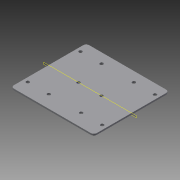
# Autodesk Inventor part: piastra_manicotti
Saved by Autodesk Inventor 2014 SP1 (Build 180222100, 222)
## iProperties
Created: 2015-04-08
Part Number: piastra_manicotti
Material: Generic
Document SubType Name: Modeling
Designer: Giorgio Nuzzo
Density: 1 g/cm^3
Appearance: Default
d2: 4,000 mm
d3: 2,000 mm
d4: 0,00 deg
d5: 4,200 mm
d6: 15,000 mm
d7: 4,200 mm
d8: 5,500 mm
d9: 12,900 mm
d10: 4,200 mm
d11: 27,400 mm
d12: 12,900 mm
d13: 2,000 mm
d14: 0,00 deg
Author: Giorgio Nuzzo
Autodesk Inventor part; units mm, degrees
ref_plane "YZ Plane" through (0, 0, 0) normal (1, 0, 0) x (0, 1, 0)
ref_plane "XZ Plane" through (0, 0, 0) normal (0, 1, 0) x (-1, 0, 0)
ref_plane "XY Plane" through (0, 0, 0) normal (0, 0, 1) x (1, 0, 0)
sketch "Sketch1" plane through (0, 0, 0) normal (0, 0, 1) x (1, 0, 0)
  line L0 (0, 69.8302) -> (0, -69.8234) construction
  line L1 (-76.7674, 0) -> (76.7472, 0) construction
  line L2 (-17.1109, 0.0005) -> (-17.1001, 0.2151)
  line L3 (-17.1001, 0.2151) -> (-17.0684, 0.4237)
  line L4 (-17.0684, 0.4237) -> (-17.0166, 0.6249)
  line L5 (-17.0166, 0.6249) -> (-16.9459, 0.8178)
  line L6 (-16.9459, 0.8178) -> (-16.8576, 1.0014)
  line L7 (-16.8576, 1.0014) -> (-16.7523, 1.1745)
  line L8 (-16.7523, 1.1745) -> (-16.6314, 1.3361)
  line L9 (-16.6314, 1.3361) -> (-16.496, 1.4853)
  line L10 (-16.496, 1.4853) -> (-16.3468, 1.6209)
  line L11 (-16.3468, 1.6209) -> (-16.1851, 1.7418)
  line L12 (-16.1851, 1.7418) -> (-16.012, 1.8469)
  line L13 (-16.012, 1.8469) -> (-15.8285, 1.9354)
  line L14 (-15.8285, 1.9354) -> (-15.6354, 2.006)
  line L15 (-15.6354, 2.006) -> (-15.4342, 2.0577)
  line L16 (-15.4342, 2.0577) -> (-15.2258, 2.0896)
  line L17 (-15.2258, 2.0896) -> (-15.011, 2.1004)
  line L18 (-15.011, 2.1004) -> (-14.7964, 2.0896)
  line L19 (-14.7964, 2.0896) -> (-14.5878, 2.0577)
  line L20 (-14.5878, 2.0577) -> (-14.3866, 2.006)
  line L21 (-14.3866, 2.006) -> (-14.1936, 1.9354)
  line L22 (-14.1936, 1.9354) -> (-14.01, 1.8469)
  line L23 (-14.01, 1.8469) -> (-13.8369, 1.7418)
  line L24 (-13.8369, 1.7418) -> (-13.6752, 1.6209)
  line L25 (-13.6752, 1.6209) -> (-13.5262, 1.4853)
  line L26 (-13.5262, 1.4853) -> (-13.3906, 1.3361)
  line L27 (-13.3906, 1.3361) -> (-13.2697, 1.1745)
  line L28 (-13.2697, 1.1745) -> (-13.1644, 1.0014)
  line L29 (-13.1644, 1.0014) -> (-13.0761, 0.8178)
  line L30 (-13.0761, 0.8178) -> (-13.0054, 0.6249)
  line L31 (-13.0054, 0.6249) -> (-12.9537, 0.4237)
  line L32 (-12.9537, 0.4237) -> (-12.9219, 0.2151)
  line L33 (-12.9219, 0.2151) -> (-12.911, 0.0005)
  line L34 (-12.911, 0.0005) -> (-12.9219, -0.2143)
  line L35 (-12.9219, -0.2143) -> (-12.9537, -0.4228)
  line L36 (-12.9537, -0.4228) -> (-13.0054, -0.624)
  line L37 (-13.0054, -0.624) -> (-13.0761, -0.8169)
  line L38 (-13.0761, -0.8169) -> (-13.1644, -1.0005)
  line L39 (-13.1644, -1.0005) -> (-13.2697, -1.1738)
  line L40 (-13.2697, -1.1738) -> (-13.3906, -1.3354)
  line L41 (-13.3906, -1.3354) -> (-13.5262, -1.4846)
  line L42 (-13.5262, -1.4846) -> (-13.6752, -1.6199)
  line L43 (-13.6752, -1.6199) -> (-13.8369, -1.7409)
  line L44 (-13.8369, -1.7409) -> (-14.01, -1.8463)
  line L45 (-14.01, -1.8463) -> (-14.1936, -1.9345)
  line L46 (-14.1936, -1.9345) -> (-14.3866, -2.0051)
  line L47 (-14.3866, -2.0051) -> (-14.5878, -2.0568)
  line L48 (-14.5878, -2.0568) -> (-14.7964, -2.0888)
  line L49 (-14.7964, -2.0888) -> (-15.011, -2.0995)
  line L50 (-15.011, -2.0995) -> (-15.2258, -2.0888)
  line L51 (-15.2258, -2.0888) -> (-15.4342, -2.0568)
  line L52 (-15.4342, -2.0568) -> (-15.6354, -2.0051)
  line L53 (-15.6354, -2.0051) -> (-15.8285, -1.9345)
  line L54 (-15.8285, -1.9345) -> (-16.012, -1.8463)
  line L55 (-16.012, -1.8463) -> (-16.1851, -1.7409)
  line L56 (-16.1851, -1.7409) -> (-16.3468, -1.6199)
  line L57 (-16.3468, -1.6199) -> (-16.496, -1.4846)
  line L58 (-16.496, -1.4846) -> (-16.6314, -1.3354)
  line L59 (-16.6314, -1.3354) -> (-16.7523, -1.1738)
  line L60 (-16.7523, -1.1738) -> (-16.8576, -1.0005)
  line L61 (-16.8576, -1.0005) -> (-16.9459, -0.8169)
  line L62 (-16.9459, -0.8169) -> (-17.0166, -0.624)
  line L63 (-17.0166, -0.624) -> (-17.0684, -0.4228)
  line L64 (-17.0684, -0.4228) -> (-17.1001, -0.2143)
  line L65 (-17.1001, -0.2143) -> (-17.1109, 0.0005)
  spline S0 degree 3 poles (-53.96, -44.9961) (-53.96, -47.2051) (-52.1691, -48.9962) (-49.9599, -48.9962) knots 0 0 0 0 1 1 1 1
  line L66 (-53.96, -44.9961) -> (-53.96, -47.2051) construction
  line L67 (-53.96, -47.2051) -> (-52.1691, -48.9962) construction
  line L68 (-52.1691, -48.9962) -> (-49.9599, -48.9962) construction
  line L69 (-49.9599, -48.9962) -> (49.9401, -48.9962)
  spline S1 degree 3 poles (49.9401, -48.9962) (52.1491, -48.9962) (53.9398, -47.2051) (53.9398, -44.9961) knots 2 2 2 2 3 3 3 3
  line L70 (49.9401, -48.9962) -> (52.1491, -48.9962) construction
  line L71 (52.1491, -48.9962) -> (53.9398, -47.2051) construction
  line L72 (53.9398, -47.2051) -> (53.9398, -44.9961) construction
  line L73 (53.9398, -44.9961) -> (53.9398, 45.0029)
  spline S2 degree 3 poles (53.9398, 45.0029) (53.9398, 47.212) (52.1491, 49.003) (49.9401, 49.003) knots 4 4 4 4 5 5 5 5
  line L74 (53.9398, 45.0029) -> (53.9398, 47.212) construction
  line L75 (53.9398, 47.212) -> (52.1491, 49.003) construction
  line L76 (52.1491, 49.003) -> (49.9401, 49.003) construction
  line L77 (49.9401, 49.003) -> (-49.9599, 49.003)
  spline S3 degree 3 poles (-49.9599, 49.003) (-52.1691, 49.003) (-53.96, 47.212) (-53.96, 45.0029) knots 6 6 6 6 7 7 7 7
  line L78 (-49.9599, 49.003) -> (-52.1691, 49.003) construction
  line L79 (-52.1691, 49.003) -> (-53.96, 47.212) construction
  line L80 (-53.96, 47.212) -> (-53.96, 45.0029) construction
  line L81 (-53.96, 45.0029) -> (-53.96, -44.9961)
  line L82 (39.7398, -16.7966) -> (39.7516, -16.5665)
  line L83 (39.7516, -16.5665) -> (39.7857, -16.3432)
  line L84 (39.7857, -16.3432) -> (39.8411, -16.1276)
  line L85 (39.8411, -16.1276) -> (39.9169, -15.9209)
  line L86 (39.9169, -15.9209) -> (40.0117, -15.7242)
  line L87 (40.0117, -15.7242) -> (40.1243, -15.5385)
  line L88 (40.1243, -15.5385) -> (40.2539, -15.3655)
  line L89 (40.2539, -15.3655) -> (40.3989, -15.2057)
  line L90 (40.3989, -15.2057) -> (40.5587, -15.0603)
  line L91 (40.5587, -15.0603) -> (40.732, -14.9308)
  line L92 (40.732, -14.9308) -> (40.9174, -14.8181)
  line L93 (40.9174, -14.8181) -> (41.1141, -14.7234)
  line L94 (41.1141, -14.7234) -> (41.3208, -14.6479)
  line L95 (41.3208, -14.6479) -> (41.5365, -14.5925)
  line L96 (41.5365, -14.5925) -> (41.7601, -14.5583)
  line L97 (41.7601, -14.5583) -> (41.9898, -14.5466)
  line L98 (41.9898, -14.5466) -> (42.22, -14.5583)
  line L99 (42.22, -14.5583) -> (42.4436, -14.5925)
  line L100 (42.4436, -14.5925) -> (42.6592, -14.6479)
  line L101 (42.6592, -14.6479) -> (42.8659, -14.7234)
  line L102 (42.8659, -14.7234) -> (43.0626, -14.8181)
  line L103 (43.0626, -14.8181) -> (43.248, -14.9308)
  line L104 (43.248, -14.9308) -> (43.4213, -15.0603)
  line L105 (43.4213, -15.0603) -> (43.5811, -15.2057)
  line L106 (43.5811, -15.2057) -> (43.7262, -15.3655)
  line L107 (43.7262, -15.3655) -> (43.8557, -15.5385)
  line L108 (43.8557, -15.5385) -> (43.9684, -15.7242)
  line L109 (43.9684, -15.7242) -> (44.0631, -15.9209)
  line L110 (44.0631, -15.9209) -> (44.1389, -16.1276)
  line L111 (44.1389, -16.1276) -> (44.1944, -16.3432)
  line L112 (44.1944, -16.3432) -> (44.2285, -16.5665)
  line L113 (44.2285, -16.5665) -> (44.2398, -16.7966)
  line L114 (44.2398, -16.7966) -> (44.2285, -17.0268)
  line L115 (44.2285, -17.0268) -> (44.1944, -17.25)
  line L116 (44.1944, -17.25) -> (44.1389, -17.4657)
  line L117 (44.1389, -17.4657) -> (44.0631, -17.6724)
  line L118 (44.0631, -17.6724) -> (43.9684, -17.8691)
  line L119 (43.9684, -17.8691) -> (43.8557, -18.0548)
  line L120 (43.8557, -18.0548) -> (43.7262, -18.2277)
  line L121 (43.7262, -18.2277) -> (43.5811, -18.3876)
  line L122 (43.5811, -18.3876) -> (43.4213, -18.533)
  line L123 (43.4213, -18.533) -> (43.248, -18.6625)
  line L124 (43.248, -18.6625) -> (43.0626, -18.7751)
  line L125 (43.0626, -18.7751) -> (42.8659, -18.8699)
  line L126 (42.8659, -18.8699) -> (42.6592, -18.9453)
  line L127 (42.6592, -18.9453) -> (42.4436, -19.0008)
  line L128 (42.4436, -19.0008) -> (42.22, -19.0349)
  line L129 (42.22, -19.0349) -> (41.9898, -19.0466)
  line L130 (41.9898, -19.0466) -> (41.7601, -19.0349)
  line L131 (41.7601, -19.0349) -> (41.5365, -19.0008)
  line L132 (41.5365, -19.0008) -> (41.3208, -18.9453)
  line L133 (41.3208, -18.9453) -> (41.1141, -18.8699)
  line L134 (41.1141, -18.8699) -> (40.9174, -18.7751)
  line L135 (40.9174, -18.7751) -> (40.732, -18.6625)
  line L136 (40.732, -18.6625) -> (40.5587, -18.533)
  line L137 (40.5587, -18.533) -> (40.3989, -18.3876)
  line L138 (40.3989, -18.3876) -> (40.2539, -18.2277)
  line L139 (40.2539, -18.2277) -> (40.1243, -18.0548)
  line L140 (40.1243, -18.0548) -> (40.0117, -17.8691)
  line L141 (40.0117, -17.8691) -> (39.9169, -17.6724)
  line L142 (39.9169, -17.6724) -> (39.8411, -17.4657)
  line L143 (39.8411, -17.4657) -> (39.7857, -17.25)
  line L144 (39.7857, -17.25) -> (39.7516, -17.0268)
  line L145 (39.7516, -17.0268) -> (39.7398, -16.7966)
  line L146 (-23.21, 36.0918) -> (-23.1986, 36.3168)
  line L147 (-23.1986, 36.3168) -> (-23.1654, 36.5352)
  line L148 (-23.1654, 36.5352) -> (-23.1111, 36.746)
  line L149 (-23.1111, 36.746) -> (-23.0372, 36.9481)
  line L150 (-23.0372, 36.9481) -> (-22.9445, 37.1405)
  line L151 (-22.9445, 37.1405) -> (-22.8343, 37.3219)
  line L152 (-22.8343, 37.3219) -> (-22.7077, 37.4912)
  line L153 (-22.7077, 37.4912) -> (-22.5656, 37.6474)
  line L154 (-22.5656, 37.6474) -> (-22.4093, 37.7894)
  line L155 (-22.4093, 37.7894) -> (-22.24, 37.916)
  line L156 (-22.24, 37.916) -> (-22.0586, 38.0262)
  line L157 (-22.0586, 38.0262) -> (-21.8664, 38.1189)
  line L158 (-21.8664, 38.1189) -> (-21.6642, 38.1928)
  line L159 (-21.6642, 38.1928) -> (-21.4533, 38.247)
  line L160 (-21.4533, 38.247) -> (-21.2349, 38.2805)
  line L161 (-21.2349, 38.2805) -> (-21.0099, 38.2918)
  line L162 (-21.0099, 38.2918) -> (-20.7851, 38.2805)
  line L163 (-20.7851, 38.2805) -> (-20.5665, 38.247)
  line L164 (-20.5665, 38.247) -> (-20.3557, 38.1928)
  line L165 (-20.3557, 38.1928) -> (-20.1537, 38.1189)
  line L166 (-20.1537, 38.1189) -> (-19.9614, 38.0262)
  line L167 (-19.9614, 38.0262) -> (-19.78, 37.916)
  line L168 (-19.78, 37.916) -> (-19.6105, 37.7894)
  line L169 (-19.6105, 37.7894) -> (-19.4543, 37.6474)
  line L170 (-19.4543, 37.6474) -> (-19.3124, 37.4912)
  line L171 (-19.3124, 37.4912) -> (-19.1858, 37.3219)
  line L172 (-19.1858, 37.3219) -> (-19.0755, 37.1405)
  line L173 (-19.0755, 37.1405) -> (-18.9828, 36.9481)
  line L174 (-18.9828, 36.9481) -> (-18.9089, 36.746)
  line L175 (-18.9089, 36.746) -> (-18.8547, 36.5352)
  line L176 (-18.8547, 36.5352) -> (-18.8214, 36.3168)
  line L177 (-18.8214, 36.3168) -> (-18.8101, 36.0918)
  line L178 (-18.8101, 36.0918) -> (-18.8214, 35.8668)
  line L179 (-18.8214, 35.8668) -> (-18.8547, 35.6484)
  line L180 (-18.8547, 35.6484) -> (-18.9089, 35.4376)
  line L181 (-18.9089, 35.4376) -> (-18.9828, 35.2353)
  line L182 (-18.9828, 35.2353) -> (-19.0755, 35.0431)
  line L183 (-19.0755, 35.0431) -> (-19.1858, 34.8617)
  line L184 (-19.1858, 34.8617) -> (-19.3124, 34.6924)
  line L185 (-19.3124, 34.6924) -> (-19.4543, 34.5362)
  line L186 (-19.4543, 34.5362) -> (-19.6105, 34.394)
  line L187 (-19.6105, 34.394) -> (-19.78, 34.2674)
  line L188 (-19.78, 34.2674) -> (-19.9614, 34.1574)
  line L189 (-19.9614, 34.1574) -> (-20.1537, 34.0647)
  line L190 (-20.1537, 34.0647) -> (-20.3557, 33.9906)
  line L191 (-20.3557, 33.9906) -> (-20.5665, 33.9365)
  line L192 (-20.5665, 33.9365) -> (-20.7851, 33.9031)
  line L193 (-20.7851, 33.9031) -> (-21.0099, 33.8918)
  line L194 (-21.0099, 33.8918) -> (-21.2349, 33.9031)
  line L195 (-21.2349, 33.9031) -> (-21.4533, 33.9365)
  line L196 (-21.4533, 33.9365) -> (-21.6642, 33.9906)
  line L197 (-21.6642, 33.9906) -> (-21.8664, 34.0647)
  line L198 (-21.8664, 34.0647) -> (-22.0586, 34.1574)
  line L199 (-22.0586, 34.1574) -> (-22.24, 34.2674)
  line L200 (-22.24, 34.2674) -> (-22.4093, 34.394)
  line L201 (-22.4093, 34.394) -> (-22.5656, 34.5362)
  line L202 (-22.5656, 34.5362) -> (-22.7077, 34.6924)
  line L203 (-22.7077, 34.6924) -> (-22.8343, 34.8617)
  line L204 (-22.8343, 34.8617) -> (-22.9445, 35.0431)
  line L205 (-22.9445, 35.0431) -> (-23.0372, 35.2353)
  line L206 (-23.0372, 35.2353) -> (-23.1111, 35.4376)
  line L207 (-23.1111, 35.4376) -> (-23.1654, 35.6484)
  line L208 (-23.1654, 35.6484) -> (-23.1986, 35.8668)
  line L209 (-23.1986, 35.8668) -> (-23.21, 36.0918)
  line L210 (18.7733, 36.0921) -> (18.7847, 36.3171)
  line L211 (18.7847, 36.3171) -> (18.8181, 36.5355)
  line L212 (18.8181, 36.5355) -> (18.8722, 36.7464)
  line L213 (18.8722, 36.7464) -> (18.9463, 36.9484)
  line L214 (18.9463, 36.9484) -> (19.039, 37.1407)
  line L215 (19.039, 37.1407) -> (19.1492, 37.322)
  line L216 (19.1492, 37.322) -> (19.2756, 37.4915)
  line L217 (19.2756, 37.4915) -> (19.4179, 37.6478)
  line L218 (19.4179, 37.6478) -> (19.574, 37.7897)
  line L219 (19.574, 37.7897) -> (19.7435, 37.9163)
  line L220 (19.7435, 37.9163) -> (19.9247, 38.0266)
  line L221 (19.9247, 38.0266) -> (20.1169, 38.1192)
  line L222 (20.1169, 38.1192) -> (20.3192, 38.1931)
  line L223 (20.3192, 38.1931) -> (20.53, 38.2474)
  line L224 (20.53, 38.2474) -> (20.7484, 38.2808)
  line L225 (20.7484, 38.2808) -> (20.9734, 38.292)
  line L226 (20.9734, 38.292) -> (21.1983, 38.2808)
  line L227 (21.1983, 38.2808) -> (21.4168, 38.2474)
  line L228 (21.4168, 38.2474) -> (21.6276, 38.1931)
  line L229 (21.6276, 38.1931) -> (21.8298, 38.1192)
  line L230 (21.8298, 38.1192) -> (22.0221, 38.0266)
  line L231 (22.0221, 38.0266) -> (22.2036, 37.9163)
  line L232 (22.2036, 37.9163) -> (22.3728, 37.7897)
  line L233 (22.3728, 37.7897) -> (22.5292, 37.6478)
  line L234 (22.5292, 37.6478) -> (22.6711, 37.4915)
  line L235 (22.6711, 37.4915) -> (22.7976, 37.322)
  line L236 (22.7976, 37.322) -> (22.9078, 37.1407)
  line L237 (22.9078, 37.1407) -> (23.0005, 36.9484)
  line L238 (23.0005, 36.9484) -> (23.0745, 36.7464)
  line L239 (23.0745, 36.7464) -> (23.1286, 36.5355)
  line L240 (23.1286, 36.5355) -> (23.162, 36.3171)
  line L241 (23.162, 36.3171) -> (23.1734, 36.0921)
  line L242 (23.1734, 36.0921) -> (23.162, 35.8672)
  line L243 (23.162, 35.8672) -> (23.1286, 35.6488)
  line L244 (23.1286, 35.6488) -> (23.0745, 35.4379)
  line L245 (23.0745, 35.4379) -> (23.0005, 35.2357)
  line L246 (23.0005, 35.2357) -> (22.9078, 35.0435)
  line L247 (22.9078, 35.0435) -> (22.7976, 34.8621)
  line L248 (22.7976, 34.8621) -> (22.6711, 34.6927)
  line L249 (22.6711, 34.6927) -> (22.5292, 34.5365)
  line L250 (22.5292, 34.5365) -> (22.3728, 34.3944)
  line L251 (22.3728, 34.3944) -> (22.2036, 34.2678)
  line L252 (22.2036, 34.2678) -> (22.0221, 34.1575)
  line L253 (22.0221, 34.1575) -> (21.8298, 34.065)
  line L254 (21.8298, 34.065) -> (21.6276, 33.991)
  line L255 (21.6276, 33.991) -> (21.4168, 33.9367)
  line L256 (21.4168, 33.9367) -> (21.1983, 33.9035)
  line L257 (21.1983, 33.9035) -> (20.9734, 33.8921)
  line L258 (20.9734, 33.8921) -> (20.7484, 33.9035)
  line L259 (20.7484, 33.9035) -> (20.53, 33.9367)
  line L260 (20.53, 33.9367) -> (20.3192, 33.991)
  line L261 (20.3192, 33.991) -> (20.1169, 34.065)
  line L262 (20.1169, 34.065) -> (19.9247, 34.1575)
  line L263 (19.9247, 34.1575) -> (19.7435, 34.2678)
  line L264 (19.7435, 34.2678) -> (19.574, 34.3944)
  line L265 (19.574, 34.3944) -> (19.4179, 34.5365)
  line L266 (19.4179, 34.5365) -> (19.2756, 34.6927)
  line L267 (19.2756, 34.6927) -> (19.1492, 34.8621)
  line L268 (19.1492, 34.8621) -> (19.039, 35.0435)
  line L269 (19.039, 35.0435) -> (18.9463, 35.2357)
  line L270 (18.9463, 35.2357) -> (18.8722, 35.4379)
  line L271 (18.8722, 35.4379) -> (18.8181, 35.6488)
  line L272 (18.8181, 35.6488) -> (18.7847, 35.8672)
  line L273 (18.7847, 35.8672) -> (18.7733, 36.0921)
  line L274 (46.1946, 36.0921) -> (46.2059, 36.3171)
  line L275 (46.2059, 36.3171) -> (46.239, 36.5355)
  line L276 (46.239, 36.5355) -> (46.2935, 36.7464)
  line L277 (46.2935, 36.7464) -> (46.3672, 36.9484)
  line L278 (46.3672, 36.9484) -> (46.4599, 37.1407)
  line L279 (46.4599, 37.1407) -> (46.5701, 37.322)
  line L280 (46.5701, 37.322) -> (46.6969, 37.4915)
  line L281 (46.6969, 37.4915) -> (46.8388, 37.6478)
  line L282 (46.8388, 37.6478) -> (46.9949, 37.7897)
  line L283 (46.9949, 37.7897) -> (47.1644, 37.9163)
  line L284 (47.1644, 37.9163) -> (47.3459, 38.0266)
  line L285 (47.3459, 38.0266) -> (47.5382, 38.1192)
  line L286 (47.5382, 38.1192) -> (47.74, 38.1931)
  line L287 (47.74, 38.1931) -> (47.9509, 38.2474)
  line L288 (47.9509, 38.2474) -> (48.1697, 38.2808)
  line L289 (48.1697, 38.2808) -> (48.3943, 38.292)
  line L290 (48.3943, 38.292) -> (48.6192, 38.2808)
  line L291 (48.6192, 38.2808) -> (48.8377, 38.2474)
  line L292 (48.8377, 38.2474) -> (49.0485, 38.1931)
  line L293 (49.0485, 38.1931) -> (49.2507, 38.1192)
  line L294 (49.2507, 38.1192) -> (49.443, 38.0266)
  line L295 (49.443, 38.0266) -> (49.6245, 37.9163)
  line L296 (49.6245, 37.9163) -> (49.7937, 37.7897)
  line L297 (49.7937, 37.7897) -> (49.9501, 37.6478)
  line L298 (49.9501, 37.6478) -> (50.092, 37.4915)
  line L299 (50.092, 37.4915) -> (50.2188, 37.322)
  line L300 (50.2188, 37.322) -> (50.329, 37.1407)
  line L301 (50.329, 37.1407) -> (50.4214, 36.9484)
  line L302 (50.4214, 36.9484) -> (50.4954, 36.7464)
  line L303 (50.4954, 36.7464) -> (50.5499, 36.5355)
  line L304 (50.5499, 36.5355) -> (50.5829, 36.3171)
  line L305 (50.5829, 36.3171) -> (50.5943, 36.0921)
  line L306 (50.5943, 36.0921) -> (50.5829, 35.8672)
  line L307 (50.5829, 35.8672) -> (50.5499, 35.6488)
  line L308 (50.5499, 35.6488) -> (50.4954, 35.4379)
  line L309 (50.4954, 35.4379) -> (50.4214, 35.2357)
  line L310 (50.4214, 35.2357) -> (50.329, 35.0435)
  line L311 (50.329, 35.0435) -> (50.2188, 34.8621)
  line L312 (50.2188, 34.8621) -> (50.092, 34.6927)
  line L313 (50.092, 34.6927) -> (49.9501, 34.5365)
  line L314 (49.9501, 34.5365) -> (49.7937, 34.3944)
  line L315 (49.7937, 34.3944) -> (49.6245, 34.2678)
  line L316 (49.6245, 34.2678) -> (49.443, 34.1575)
  line L317 (49.443, 34.1575) -> (49.2507, 34.065)
  line L318 (49.2507, 34.065) -> (49.0485, 33.991)
  line L319 (49.0485, 33.991) -> (48.8377, 33.9367)
  line L320 (48.8377, 33.9367) -> (48.6192, 33.9035)
  line L321 (48.6192, 33.9035) -> (48.3943, 33.8921)
  line L322 (48.3943, 33.8921) -> (48.1697, 33.9035)
  line L323 (48.1697, 33.9035) -> (47.9509, 33.9367)
  line L324 (47.9509, 33.9367) -> (47.74, 33.991)
  line L325 (47.74, 33.991) -> (47.5382, 34.065)
  line L326 (47.5382, 34.065) -> (47.3459, 34.1575)
  line L327 (47.3459, 34.1575) -> (47.1644, 34.2678)
  line L328 (47.1644, 34.2678) -> (46.9949, 34.3944)
  line L329 (46.9949, 34.3944) -> (46.8388, 34.5365)
  line L330 (46.8388, 34.5365) -> (46.6969, 34.6927)
  line L331 (46.6969, 34.6927) -> (46.5701, 34.8621)
  line L332 (46.5701, 34.8621) -> (46.4599, 35.0435)
  line L333 (46.4599, 35.0435) -> (46.3672, 35.2357)
  line L334 (46.3672, 35.2357) -> (46.2935, 35.4379)
  line L335 (46.2935, 35.4379) -> (46.239, 35.6488)
  line L336 (46.239, 35.6488) -> (46.2059, 35.8672)
  line L337 (46.2059, 35.8672) -> (46.1946, 36.0921)
  line L338 (12.8902, 0.0005) -> (12.9008, 0.2151)
  line L339 (12.9008, 0.2151) -> (12.9325, 0.4237)
  line L340 (12.9325, 0.4237) -> (12.9845, 0.6249)
  line L341 (12.9845, 0.6249) -> (13.0552, 0.8178)
  line L342 (13.0552, 0.8178) -> (13.1434, 1.0014)
  line L343 (13.1434, 1.0014) -> (13.2488, 1.1745)
  line L344 (13.2488, 1.1745) -> (13.3694, 1.3361)
  line L345 (13.3694, 1.3361) -> (13.5051, 1.4853)
  line L346 (13.5051, 1.4853) -> (13.6543, 1.6209)
  line L347 (13.6543, 1.6209) -> (13.8158, 1.7418)
  line L348 (13.8158, 1.7418) -> (13.9891, 1.8469)
  line L349 (13.9891, 1.8469) -> (14.1724, 1.9354)
  line L350 (14.1724, 1.9354) -> (14.3657, 2.006)
  line L351 (14.3657, 2.006) -> (14.5669, 2.0577)
  line L352 (14.5669, 2.0577) -> (14.7753, 2.0896)
  line L353 (14.7753, 2.0896) -> (14.9899, 2.1004)
  line L354 (14.9899, 2.1004) -> (15.2046, 2.0896)
  line L355 (15.2046, 2.0896) -> (15.4133, 2.0577)
  line L356 (15.4133, 2.0577) -> (15.6145, 2.006)
  line L357 (15.6145, 2.006) -> (15.8075, 1.9354)
  line L358 (15.8075, 1.9354) -> (15.9911, 1.8469)
  line L359 (15.9911, 1.8469) -> (16.164, 1.7418)
  line L360 (16.164, 1.7418) -> (16.3259, 1.6209)
  line L361 (16.3259, 1.6209) -> (16.4748, 1.4853)
  line L362 (16.4748, 1.4853) -> (16.6105, 1.3361)
  line L363 (16.6105, 1.3361) -> (16.7314, 1.1745)
  line L364 (16.7314, 1.1745) -> (16.8365, 1.0014)
  line L365 (16.8365, 1.0014) -> (16.925, 0.8178)
  line L366 (16.925, 0.8178) -> (16.9957, 0.6249)
  line L367 (16.9957, 0.6249) -> (17.0473, 0.4237)
  line L368 (17.0473, 0.4237) -> (17.079, 0.2151)
  line L369 (17.079, 0.2151) -> (17.0901, 0.0005)
  line L370 (17.0901, 0.0005) -> (17.079, -0.2143)
  line L371 (17.079, -0.2143) -> (17.0473, -0.4228)
  line L372 (17.0473, -0.4228) -> (16.9957, -0.624)
  line L373 (16.9957, -0.624) -> (16.925, -0.8169)
  line L374 (16.925, -0.8169) -> (16.8365, -1.0005)
  line L375 (16.8365, -1.0005) -> (16.7314, -1.1738)
  line L376 (16.7314, -1.1738) -> (16.6105, -1.3354)
  line L377 (16.6105, -1.3354) -> (16.4748, -1.4846)
  line L378 (16.4748, -1.4846) -> (16.3259, -1.6199)
  line L379 (16.3259, -1.6199) -> (16.164, -1.7409)
  line L380 (16.164, -1.7409) -> (15.9911, -1.8463)
  line L381 (15.9911, -1.8463) -> (15.8075, -1.9345)
  line L382 (15.8075, -1.9345) -> (15.6145, -2.0051)
  line L383 (15.6145, -2.0051) -> (15.4133, -2.0568)
  line L384 (15.4133, -2.0568) -> (15.2046, -2.0888)
  line L385 (15.2046, -2.0888) -> (14.9899, -2.0995)
  line L386 (14.9899, -2.0995) -> (14.7753, -2.0888)
  line L387 (14.7753, -2.0888) -> (14.5669, -2.0568)
  line L388 (14.5669, -2.0568) -> (14.3657, -2.0051)
  line L389 (14.3657, -2.0051) -> (14.1724, -1.9345)
  line L390 (14.1724, -1.9345) -> (13.9891, -1.8463)
  line L391 (13.9891, -1.8463) -> (13.8158, -1.7409)
  line L392 (13.8158, -1.7409) -> (13.6543, -1.6199)
  line L393 (13.6543, -1.6199) -> (13.5051, -1.4846)
  line L394 (13.5051, -1.4846) -> (13.3694, -1.3354)
  line L395 (13.3694, -1.3354) -> (13.2488, -1.1738)
  line L396 (13.2488, -1.1738) -> (13.1434, -1.0005)
  line L397 (13.1434, -1.0005) -> (13.0552, -0.8169)
  line L398 (13.0552, -0.8169) -> (12.9845, -0.624)
  line L399 (12.9845, -0.624) -> (12.9325, -0.4228)
  line L400 (12.9325, -0.4228) -> (12.9008, -0.2143)
  line L401 (12.9008, -0.2143) -> (12.8902, 0.0005)
  line L402 (46.1946, -32.6403) -> (46.2059, -32.4153)
  line L403 (46.2059, -32.4153) -> (46.239, -32.1969)
  line L404 (46.239, -32.1969) -> (46.2935, -31.986)
  line L405 (46.2935, -31.986) -> (46.3672, -31.7838)
  line L406 (46.3672, -31.7838) -> (46.4599, -31.5916)
  line L407 (46.4599, -31.5916) -> (46.5701, -31.41)
  line L408 (46.5701, -31.41) -> (46.6969, -31.2409)
  line L409 (46.6969, -31.2409) -> (46.8388, -31.0845)
  line L410 (46.8388, -31.0845) -> (46.9949, -30.9425)
  line L411 (46.9949, -30.9425) -> (47.1644, -30.8161)
  line L412 (47.1644, -30.8161) -> (47.3459, -30.7059)
  line L413 (47.3459, -30.7059) -> (47.5382, -30.6132)
  line L414 (47.5382, -30.6132) -> (47.74, -30.5391)
  line L415 (47.74, -30.5391) -> (47.9509, -30.485)
  line L416 (47.9509, -30.485) -> (48.1697, -30.4516)
  line L417 (48.1697, -30.4516) -> (48.3943, -30.4402)
  line L418 (48.3943, -30.4402) -> (48.6192, -30.4516)
  line L419 (48.6192, -30.4516) -> (48.8377, -30.485)
  line L420 (48.8377, -30.485) -> (49.0485, -30.5391)
  line L421 (49.0485, -30.5391) -> (49.2507, -30.6132)
  line L422 (49.2507, -30.6132) -> (49.443, -30.7059)
  line L423 (49.443, -30.7059) -> (49.6245, -30.8161)
  line L424 (49.6245, -30.8161) -> (49.7937, -30.9425)
  line L425 (49.7937, -30.9425) -> (49.9501, -31.0845)
  line L426 (49.9501, -31.0845) -> (50.092, -31.2409)
  line L427 (50.092, -31.2409) -> (50.2188, -31.41)
  line L428 (50.2188, -31.41) -> (50.329, -31.5916)
  line L429 (50.329, -31.5916) -> (50.4214, -31.7838)
  line L430 (50.4214, -31.7838) -> (50.4954, -31.986)
  line L431 (50.4954, -31.986) -> (50.5499, -32.1969)
  line L432 (50.5499, -32.1969) -> (50.5829, -32.4153)
  line L433 (50.5829, -32.4153) -> (50.5943, -32.6403)
  line L434 (50.5943, -32.6403) -> (50.5829, -32.8652)
  line L435 (50.5829, -32.8652) -> (50.5499, -33.0837)
  line L436 (50.5499, -33.0837) -> (50.4954, -33.2945)
  line L437 (50.4954, -33.2945) -> (50.4214, -33.4967)
  line L438 (50.4214, -33.4967) -> (50.329, -33.689)
  line L439 (50.329, -33.689) -> (50.2188, -33.8702)
  line L440 (50.2188, -33.8702) -> (50.092, -34.0397)
  line L441 (50.092, -34.0397) -> (49.9501, -34.1957)
  line L442 (49.9501, -34.1957) -> (49.7937, -34.338)
  line L443 (49.7937, -34.338) -> (49.6245, -34.4645)
  line L444 (49.6245, -34.4645) -> (49.443, -34.5747)
  line L445 (49.443, -34.5747) -> (49.2507, -34.6674)
  line L446 (49.2507, -34.6674) -> (49.0485, -34.7414)
  line L447 (49.0485, -34.7414) -> (48.8377, -34.7955)
  line L448 (48.8377, -34.7955) -> (48.6192, -34.8289)
  line L449 (48.6192, -34.8289) -> (48.3943, -34.8403)
  line L450 (48.3943, -34.8403) -> (48.1697, -34.8289)
  line L451 (48.1697, -34.8289) -> (47.9509, -34.7955)
  line L452 (47.9509, -34.7955) -> (47.74, -34.7414)
  line L453 (47.74, -34.7414) -> (47.5382, -34.6674)
  line L454 (47.5382, -34.6674) -> (47.3459, -34.5747)
  line L455 (47.3459, -34.5747) -> (47.1644, -34.4645)
  line L456 (47.1644, -34.4645) -> (46.9949, -34.338)
  line L457 (46.9949, -34.338) -> (46.8388, -34.1957)
  line L458 (46.8388, -34.1957) -> (46.6969, -34.0397)
  line L459 (46.6969, -34.0397) -> (46.5701, -33.8702)
  line L460 (46.5701, -33.8702) -> (46.4599, -33.689)
  line L461 (46.4599, -33.689) -> (46.3672, -33.4967)
  line L462 (46.3672, -33.4967) -> (46.2935, -33.2945)
  line L463 (46.2935, -33.2945) -> (46.239, -33.0837)
  line L464 (46.239, -33.0837) -> (46.2059, -32.8652)
  line L465 (46.2059, -32.8652) -> (46.1946, -32.6403)
  line L466 (18.7733, -32.6406) -> (18.7847, -32.4157)
  line L467 (18.7847, -32.4157) -> (18.8181, -32.1972)
  line L468 (18.8181, -32.1972) -> (18.8722, -31.9864)
  line L469 (18.8722, -31.9864) -> (18.9463, -31.7842)
  line L470 (18.9463, -31.7842) -> (19.039, -31.5919)
  line L471 (19.039, -31.5919) -> (19.1492, -31.4104)
  line L472 (19.1492, -31.4104) -> (19.2756, -31.2412)
  line L473 (19.2756, -31.2412) -> (19.4179, -31.0848)
  line L474 (19.4179, -31.0848) -> (19.574, -30.9429)
  line L475 (19.574, -30.9429) -> (19.7435, -30.8161)
  line L476 (19.7435, -30.8161) -> (19.9247, -30.7062)
  line L477 (19.9247, -30.7062) -> (20.1169, -30.6135)
  line L478 (20.1169, -30.6135) -> (20.3192, -30.5395)
  line L479 (20.3192, -30.5395) -> (20.53, -30.4854)
  line L480 (20.53, -30.4854) -> (20.7484, -30.4519)
  line L481 (20.7484, -30.4519) -> (20.9734, -30.4406)
  line L482 (20.9734, -30.4406) -> (21.1983, -30.4519)
  line L483 (21.1983, -30.4519) -> (21.4168, -30.4854)
  line L484 (21.4168, -30.4854) -> (21.6276, -30.5395)
  line L485 (21.6276, -30.5395) -> (21.8298, -30.6135)
  line L486 (21.8298, -30.6135) -> (22.0221, -30.7062)
  line L487 (22.0221, -30.7062) -> (22.2036, -30.8161)
  line L488 (22.2036, -30.8161) -> (22.3728, -30.9429)
  line L489 (22.3728, -30.9429) -> (22.5292, -31.0848)
  line L490 (22.5292, -31.0848) -> (22.6711, -31.2412)
  line L491 (22.6711, -31.2412) -> (22.7976, -31.4104)
  line L492 (22.7976, -31.4104) -> (22.9078, -31.5919)
  line L493 (22.9078, -31.5919) -> (23.0005, -31.7842)
  line L494 (23.0005, -31.7842) -> (23.0745, -31.9864)
  line L495 (23.0745, -31.9864) -> (23.1286, -32.1972)
  line L496 (23.1286, -32.1972) -> (23.162, -32.4157)
  line L497 (23.162, -32.4157) -> (23.1734, -32.6406)
  line L498 (23.1734, -32.6406) -> (23.162, -32.8656)
  line L499 (23.162, -32.8656) -> (23.1286, -33.084)
  line L500 (23.1286, -33.084) -> (23.0745, -33.2948)
  line L501 (23.0745, -33.2948) -> (23.0005, -33.4967)
  line L502 (23.0005, -33.4967) -> (22.9078, -33.6893)
  line L503 (22.9078, -33.6893) -> (22.7976, -33.8705)
  line L504 (22.7976, -33.8705) -> (22.6711, -34.04)
  line L505 (22.6711, -34.04) -> (22.5292, -34.1961)
  line L506 (22.5292, -34.1961) -> (22.3728, -34.338)
  line L507 (22.3728, -34.338) -> (22.2036, -34.4648)
  line L508 (22.2036, -34.4648) -> (22.0221, -34.575)
  line L509 (22.0221, -34.575) -> (21.8298, -34.6677)
  line L510 (21.8298, -34.6677) -> (21.6276, -34.7418)
  line L511 (21.6276, -34.7418) -> (21.4168, -34.7959)
  line L512 (21.4168, -34.7959) -> (21.1983, -34.8293)
  line L513 (21.1983, -34.8293) -> (20.9734, -34.8407)
  line L514 (20.9734, -34.8407) -> (20.7484, -34.8293)
  line L515 (20.7484, -34.8293) -> (20.53, -34.7959)
  line L516 (20.53, -34.7959) -> (20.3192, -34.7418)
  line L517 (20.3192, -34.7418) -> (20.1169, -34.6677)
  line L518 (20.1169, -34.6677) -> (19.9247, -34.575)
  line L519 (19.9247, -34.575) -> (19.7435, -34.4648)
  line L520 (19.7435, -34.4648) -> (19.574, -34.338)
  line L521 (19.574, -34.338) -> (19.4179, -34.1961)
  line L522 (19.4179, -34.1961) -> (19.2756, -34.04)
  line L523 (19.2756, -34.04) -> (19.1492, -33.8705)
  line L524 (19.1492, -33.8705) -> (19.039, -33.6893)
  line L525 (19.039, -33.6893) -> (18.9463, -33.4967)
  line L526 (18.9463, -33.4967) -> (18.8722, -33.2948)
  line L527 (18.8722, -33.2948) -> (18.8181, -33.084)
  line L528 (18.8181, -33.084) -> (18.7847, -32.8656)
  line L529 (18.7847, -32.8656) -> (18.7733, -32.6406)
  line L530 (-23.21, -32.641) -> (-23.1986, -32.416)
  line L531 (-23.1986, -32.416) -> (-23.1654, -32.1976)
  line L532 (-23.1654, -32.1976) -> (-23.1111, -31.9867)
  line L533 (-23.1111, -31.9867) -> (-23.0372, -31.7845)
  line L534 (-23.0372, -31.7845) -> (-22.9445, -31.5923)
  line L535 (-22.9445, -31.5923) -> (-22.8343, -31.4111)
  line L536 (-22.8343, -31.4111) -> (-22.7077, -31.2416)
  line L537 (-22.7077, -31.2416) -> (-22.5656, -31.0855)
  line L538 (-22.5656, -31.0855) -> (-22.4093, -30.9432)
  line L539 (-22.4093, -30.9432) -> (-22.24, -30.8168)
  line L540 (-22.24, -30.8168) -> (-22.0586, -30.7065)
  line L541 (-22.0586, -30.7065) -> (-21.8664, -30.6139)
  line L542 (-21.8664, -30.6139) -> (-21.6642, -30.5398)
  line L543 (-21.6642, -30.5398) -> (-21.4533, -30.4857)
  line L544 (-21.4533, -30.4857) -> (-21.2349, -30.4523)
  line L545 (-21.2349, -30.4523) -> (-21.0099, -30.4409)
  line L546 (-21.0099, -30.4409) -> (-20.7851, -30.4523)
  line L547 (-20.7851, -30.4523) -> (-20.5665, -30.4857)
  line L548 (-20.5665, -30.4857) -> (-20.3557, -30.5398)
  line L549 (-20.3557, -30.5398) -> (-20.1537, -30.6139)
  line L550 (-20.1537, -30.6139) -> (-19.9614, -30.7065)
  line L551 (-19.9614, -30.7065) -> (-19.78, -30.8168)
  line L552 (-19.78, -30.8168) -> (-19.6105, -30.9432)
  line L553 (-19.6105, -30.9432) -> (-19.4543, -31.0855)
  line L554 (-19.4543, -31.0855) -> (-19.3124, -31.2416)
  line L555 (-19.3124, -31.2416) -> (-19.1858, -31.4111)
  line L556 (-19.1858, -31.4111) -> (-19.0755, -31.5923)
  line L557 (-19.0755, -31.5923) -> (-18.9828, -31.7845)
  line L558 (-18.9828, -31.7845) -> (-18.9089, -31.9867)
  line L559 (-18.9089, -31.9867) -> (-18.8547, -32.1976)
  line L560 (-18.8547, -32.1976) -> (-18.8214, -32.416)
  line L561 (-18.8214, -32.416) -> (-18.8101, -32.641)
  line L562 (-18.8101, -32.641) -> (-18.8214, -32.8659)
  line L563 (-18.8214, -32.8659) -> (-18.8547, -33.0843)
  line L564 (-18.8547, -33.0843) -> (-18.9089, -33.2952)
  line L565 (-18.9089, -33.2952) -> (-18.9828, -33.4974)
  line L566 (-18.9828, -33.4974) -> (-19.0755, -33.6896)
  line L567 (-19.0755, -33.6896) -> (-19.1858, -33.8709)
  line L568 (-19.1858, -33.8709) -> (-19.3124, -34.0404)
  line L569 (-19.3124, -34.0404) -> (-19.4543, -34.1968)
  line L570 (-19.4543, -34.1968) -> (-19.6105, -34.3387)
  line L571 (-19.6105, -34.3387) -> (-19.78, -34.4651)
  line L572 (-19.78, -34.4651) -> (-19.9614, -34.5754)
  line L573 (-19.9614, -34.5754) -> (-20.1537, -34.6681)
  line L574 (-20.1537, -34.6681) -> (-20.3557, -34.7421)
  line L575 (-20.3557, -34.7421) -> (-20.5665, -34.7962)
  line L576 (-20.5665, -34.7962) -> (-20.7851, -34.8296)
  line L577 (-20.7851, -34.8296) -> (-21.0099, -34.841)
  line L578 (-21.0099, -34.841) -> (-21.2349, -34.8296)
  line L579 (-21.2349, -34.8296) -> (-21.4533, -34.7962)
  line L580 (-21.4533, -34.7962) -> (-21.6642, -34.7421)
  line L581 (-21.6642, -34.7421) -> (-21.8664, -34.6681)
  line L582 (-21.8664, -34.6681) -> (-22.0586, -34.5754)
  line L583 (-22.0586, -34.5754) -> (-22.24, -34.4651)
  line L584 (-22.24, -34.4651) -> (-22.4093, -34.3387)
  line L585 (-22.4093, -34.3387) -> (-22.5656, -34.1968)
  line L586 (-22.5656, -34.1968) -> (-22.7077, -34.0404)
  line L587 (-22.7077, -34.0404) -> (-22.8343, -33.8709)
  line L588 (-22.8343, -33.8709) -> (-22.9445, -33.6896)
  line L589 (-22.9445, -33.6896) -> (-23.0372, -33.4974)
  line L590 (-23.0372, -33.4974) -> (-23.1111, -33.2952)
  line L591 (-23.1111, -33.2952) -> (-23.1654, -33.0843)
  line L592 (-23.1654, -33.0843) -> (-23.1986, -32.8659)
  line L593 (-23.1986, -32.8659) -> (-23.21, -32.641)
  line L594 (-50.631, -32.641) -> (-50.6197, -32.416)
  line L595 (-50.6197, -32.416) -> (-50.5862, -32.1976)
  line L596 (-50.5862, -32.1976) -> (-50.5322, -31.9867)
  line L597 (-50.5322, -31.9867) -> (-50.4581, -31.7845)
  line L598 (-50.4581, -31.7845) -> (-50.3654, -31.5923)
  line L599 (-50.3654, -31.5923) -> (-50.2553, -31.4111)
  line L600 (-50.2553, -31.4111) -> (-50.1286, -31.2416)
  line L601 (-50.1286, -31.2416) -> (-49.9866, -31.0855)
  line L602 (-49.9866, -31.0855) -> (-49.8304, -30.9432)
  line L603 (-49.8304, -30.9432) -> (-49.6611, -30.8168)
  line L604 (-49.6611, -30.8168) -> (-49.4797, -30.7065)
  line L605 (-49.4797, -30.7065) -> (-49.2873, -30.6139)
  line L606 (-49.2873, -30.6139) -> (-49.0852, -30.5398)
  line L607 (-49.0852, -30.5398) -> (-48.8744, -30.4857)
  line L608 (-48.8744, -30.4857) -> (-48.656, -30.4523)
  line L609 (-48.656, -30.4523) -> (-48.431, -30.4409)
  line L610 (-48.431, -30.4409) -> (-48.206, -30.4523)
  line L611 (-48.206, -30.4523) -> (-47.9876, -30.4857)
  line L612 (-47.9876, -30.4857) -> (-47.7768, -30.5398)
  line L613 (-47.7768, -30.5398) -> (-47.5747, -30.6139)
  line L614 (-47.5747, -30.6139) -> (-47.3823, -30.7065)
  line L615 (-47.3823, -30.7065) -> (-47.2009, -30.8168)
  line L616 (-47.2009, -30.8168) -> (-47.0316, -30.9432)
  line L617 (-47.0316, -30.9432) -> (-46.8754, -31.0855)
  line L618 (-46.8754, -31.0855) -> (-46.7334, -31.2416)
  line L619 (-46.7334, -31.2416) -> (-46.6066, -31.4111)
  line L620 (-46.6066, -31.4111) -> (-46.4966, -31.5923)
  line L621 (-46.4966, -31.5923) -> (-46.4039, -31.7845)
  line L622 (-46.4039, -31.7845) -> (-46.3298, -31.9867)
  line L623 (-46.3298, -31.9867) -> (-46.2757, -32.1976)
  line L624 (-46.2757, -32.1976) -> (-46.2423, -32.416)
  line L625 (-46.2423, -32.416) -> (-46.231, -32.641)
  line L626 (-46.231, -32.641) -> (-46.2423, -32.8659)
  line L627 (-46.2423, -32.8659) -> (-46.2757, -33.0843)
  line L628 (-46.2757, -33.0843) -> (-46.3298, -33.2952)
  line L629 (-46.3298, -33.2952) -> (-46.4039, -33.4974)
  line L630 (-46.4039, -33.4974) -> (-46.4966, -33.6896)
  line L631 (-46.4966, -33.6896) -> (-46.6066, -33.8709)
  line L632 (-46.6066, -33.8709) -> (-46.7334, -34.0404)
  line L633 (-46.7334, -34.0404) -> (-46.8754, -34.1968)
  line L634 (-46.8754, -34.1968) -> (-47.0316, -34.3387)
  line L635 (-47.0316, -34.3387) -> (-47.2009, -34.4651)
  line L636 (-47.2009, -34.4651) -> (-47.3823, -34.5754)
  line L637 (-47.3823, -34.5754) -> (-47.5747, -34.6681)
  line L638 (-47.5747, -34.6681) -> (-47.7768, -34.7421)
  line L639 (-47.7768, -34.7421) -> (-47.9876, -34.7962)
  line L640 (-47.9876, -34.7962) -> (-48.206, -34.8296)
  line L641 (-48.206, -34.8296) -> (-48.431, -34.841)
  line L642 (-48.431, -34.841) -> (-48.656, -34.8296)
  line L643 (-48.656, -34.8296) -> (-48.8744, -34.7962)
  line L644 (-48.8744, -34.7962) -> (-49.0852, -34.7421)
  line L645 (-49.0852, -34.7421) -> (-49.2873, -34.6681)
  line L646 (-49.2873, -34.6681) -> (-49.4797, -34.5754)
  line L647 (-49.4797, -34.5754) -> (-49.6611, -34.4651)
  line L648 (-49.6611, -34.4651) -> (-49.8304, -34.3387)
  line L649 (-49.8304, -34.3387) -> (-49.9866, -34.1968)
  line L650 (-49.9866, -34.1968) -> (-50.1286, -34.0404)
  line L651 (-50.1286, -34.0404) -> (-50.2553, -33.8709)
  line L652 (-50.2553, -33.8709) -> (-50.3654, -33.6896)
  line L653 (-50.3654, -33.6896) -> (-50.4581, -33.4974)
  line L654 (-50.4581, -33.4974) -> (-50.5322, -33.2952)
  line L655 (-50.5322, -33.2952) -> (-50.5862, -33.0843)
  line L656 (-50.5862, -33.0843) -> (-50.6197, -32.8659)
  line L657 (-50.6197, -32.8659) -> (-50.631, -32.641)
  line L658 (-50.631, 36.0918) -> (-50.6197, 35.8668)
  line L659 (-50.6197, 35.8668) -> (-50.5862, 35.6484)
  line L660 (-50.5862, 35.6484) -> (-50.5322, 35.4376)
  line L661 (-50.5322, 35.4376) -> (-50.4581, 35.2353)
  line L662 (-50.4581, 35.2353) -> (-50.3654, 35.0431)
  line L663 (-50.3654, 35.0431) -> (-50.2553, 34.8617)
  line L664 (-50.2553, 34.8617) -> (-50.1286, 34.6924)
  line L665 (-50.1286, 34.6924) -> (-49.9866, 34.5362)
  line L666 (-49.9866, 34.5362) -> (-49.8304, 34.394)
  line L667 (-49.8304, 34.394) -> (-49.6611, 34.2674)
  line L668 (-49.6611, 34.2674) -> (-49.4797, 34.1574)
  line L669 (-49.4797, 34.1574) -> (-49.2873, 34.0647)
  line L670 (-49.2873, 34.0647) -> (-49.0852, 33.9906)
  line L671 (-49.0852, 33.9906) -> (-48.8744, 33.9365)
  line L672 (-48.8744, 33.9365) -> (-48.656, 33.9031)
  line L673 (-48.656, 33.9031) -> (-48.431, 33.8918)
  line L674 (-48.431, 33.8918) -> (-48.206, 33.9031)
  line L675 (-48.206, 33.9031) -> (-47.9876, 33.9365)
  line L676 (-47.9876, 33.9365) -> (-47.7768, 33.9906)
  line L677 (-47.7768, 33.9906) -> (-47.5747, 34.0647)
  line L678 (-47.5747, 34.0647) -> (-47.3823, 34.1574)
  line L679 (-47.3823, 34.1574) -> (-47.2009, 34.2674)
  line L680 (-47.2009, 34.2674) -> (-47.0316, 34.394)
  line L681 (-47.0316, 34.394) -> (-46.8754, 34.5362)
  line L682 (-46.8754, 34.5362) -> (-46.7334, 34.6924)
  line L683 (-46.7334, 34.6924) -> (-46.6066, 34.8617)
  line L684 (-46.6066, 34.8617) -> (-46.4966, 35.0431)
  line L685 (-46.4966, 35.0431) -> (-46.4039, 35.2353)
  line L686 (-46.4039, 35.2353) -> (-46.3298, 35.4376)
  line L687 (-46.3298, 35.4376) -> (-46.2757, 35.6484)
  line L688 (-46.2757, 35.6484) -> (-46.2423, 35.8668)
  line L689 (-46.2423, 35.8668) -> (-46.231, 36.0918)
  line L690 (-46.231, 36.0918) -> (-46.2423, 36.3168)
  line L691 (-46.2423, 36.3168) -> (-46.2757, 36.5352)
  line L692 (-46.2757, 36.5352) -> (-46.3298, 36.746)
  line L693 (-46.3298, 36.746) -> (-46.4039, 36.9481)
  line L694 (-46.4039, 36.9481) -> (-46.4966, 37.1405)
  line L695 (-46.4966, 37.1405) -> (-46.6066, 37.3219)
  line L696 (-46.6066, 37.3219) -> (-46.7334, 37.4912)
  line L697 (-46.7334, 37.4912) -> (-46.8754, 37.6474)
  line L698 (-46.8754, 37.6474) -> (-47.0316, 37.7894)
  line L699 (-47.0316, 37.7894) -> (-47.2009, 37.916)
  line L700 (-47.2009, 37.916) -> (-47.3823, 38.0262)
  line L701 (-47.3823, 38.0262) -> (-47.5747, 38.1189)
  line L702 (-47.5747, 38.1189) -> (-47.7768, 38.1928)
  line L703 (-47.7768, 38.1928) -> (-47.9876, 38.247)
  line L704 (-47.9876, 38.247) -> (-48.206, 38.2805)
  line L705 (-48.206, 38.2805) -> (-48.431, 38.2918)
  line L706 (-48.431, 38.2918) -> (-48.656, 38.2805)
  line L707 (-48.656, 38.2805) -> (-48.8744, 38.247)
  line L708 (-48.8744, 38.247) -> (-49.0852, 38.1928)
  line L709 (-49.0852, 38.1928) -> (-49.2873, 38.1189)
  line L710 (-49.2873, 38.1189) -> (-49.4797, 38.0262)
  line L711 (-49.4797, 38.0262) -> (-49.6611, 37.916)
  line L712 (-49.6611, 37.916) -> (-49.8304, 37.7894)
  line L713 (-49.8304, 37.7894) -> (-49.9866, 37.6474)
  line L714 (-49.9866, 37.6474) -> (-50.1286, 37.4912)
  line L715 (-50.1286, 37.4912) -> (-50.2553, 37.3219)
  line L716 (-50.2553, 37.3219) -> (-50.3654, 37.1405)
  line L717 (-50.3654, 37.1405) -> (-50.4581, 36.9481)
  line L718 (-50.4581, 36.9481) -> (-50.5322, 36.746)
  line L719 (-50.5322, 36.746) -> (-50.5862, 36.5352)
  line L720 (-50.5862, 36.5352) -> (-50.6197, 36.3168)
  line L721 (-50.6197, 36.3168) -> (-50.631, 36.0918)
  line L722 (-53.96, 0.0034) -> (53.9398, 0.0034) construction
  line L723 (-0.0099, 49.003) -> (-0.0099, -48.9962) construction
  point P0 (-0.0099, 0.0034)
  constraints: 1420 end point, 5 midpoint, 12 other
sketch "Sketch2" plane through (0, 0, 0) normal (0, 0, 1) x (1, 0, 0)
  line L0 (49.9401, 49.003) -> (-49.9599, 49.003) construction
  line L1 (-53.96, 45.0029) -> (-53.96, -44.9961) construction
  line L2 (-49.9599, -48.9962) -> (49.9401, -48.9962) construction
  line L3 (53.9398, -44.9961) -> (53.9398, 45.0029) construction
  line L4 (-49.96, 49.003) -> (49.9398, 49.003)
  line L5 (53.9398, 45.003) -> (53.9398, -44.9962)
  line L6 (49.9398, -48.9962) -> (-49.96, -48.9962)
  line L7 (-53.96, -44.9962) -> (-53.96, 45.003)
  arc A0 (49.9398, -48.9962) -> (53.9398, -44.9962) centre (49.9398, -44.9962) ccw
  arc A1 (-53.96, -44.9962) -> (-49.96, -48.9962) centre (-49.96, -44.9962) ccw
  arc A2 (-49.96, 49.003) -> (-53.96, 45.003) centre (-49.96, 45.003) ccw
  arc A3 (53.9398, 45.003) -> (49.9398, 49.003) centre (49.9398, 45.003) ccw
  point P0 (0, 0)
  dimension "d2" = 4
  constraints: 8 end point, 8 point on circle, 8 tangent, 4 centre point, 3 equal radius, 2 parallel, 1 horizontal, 1 perpendicular
  measures "d2" radius of A0
extrude "Extrusion1" add sketch "Sketch2" along normal blind 2
sketch "Sketch3" plane through (0, 0, 0) normal (0, 0, -1) x (-1, 0, 0)
  line L0 (-53.9398, -44.9962) -> (-53.9398, 45.003) projected
  line L1 (-49.9398, 49.003) -> (49.96, 49.003) projected
  circle A0 centre (-15, 0) radius 2.1
  line L2 (76.7674, 0) -> (-76.7472, 0) construction
  line L3 (0, 69.8302) -> (0, -69.8234) construction
  circle A1 centre (-48.4398, 36.103) radius 2.1
  circle A2 centre (-21.0398, 36.103) radius 2.1
  circle A3 centre (48.4398, 36.103) radius 2.1
  circle A4 centre (21.0398, 36.103) radius 2.1
  circle A5 centre (-48.4398, -32.5163) radius 2.1
  circle A6 centre (-21.0398, -32.5163) radius 2.1
  circle A7 centre (21.0398, -32.5163) radius 2.1
  circle A8 centre (48.4398, -32.5163) radius 2.1
  circle A9 centre (15, 0) radius 2.1
  point P0 (0, 0)
  dimension "d5" = 4.2
  dimension "d6" = 15
  dimension "d7" = 4.2
  dimension "d8" = 5.5
  dimension "d9" = 12.9
  dimension "d10" = 4.2
  dimension "d11" = 27.4
  dimension "d12" = 12.9
  constraints: 10 centre point, 3 symmetric about line, 1 point on line, 3 other
  measures "d5" diameter of A0
  measures "d6" distance from line of L3 A0.centre
  measures "d7" diameter of A1
  measures "d8" distance from line of L0 A1.centre
  measures "d9" distance from line of L1 A1.centre
  measures "d10" diameter of A2
  measures "d11" distance of A2.centre A1.centre
  measures "d12" distance from line of L1 A2.centre
extrude "Extrusion2" cut sketch "Sketch3" against normal blind 2
ref_plane "Work Plane1" through (-49.96, 0.0034, 0) normal (0, 1, 0) x (1, 0, 0)
equation "\"d10\" = d7"
equation "\"d12\" = d9"
body "Solid1"
